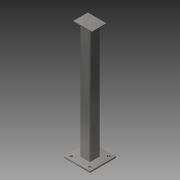
# Autodesk Inventor part: Ст1 - Metal rack
Saved by Autodesk Inventor 2020.1 (Build 241239000, 239)
## iProperties
Created: 2017-07-27
Part Number: Ст1 - Metal rack
Material: Сталь, углеродистая
Document SubType Name: Modeling
Designer: Головченко
Density: 7.87 g/cm^3
Appearance: Сталь — полированная
Mass&: 0
Author: Головченко
Autodesk Inventor part; units mm, degrees
(part 1 of 4)
ref_plane "YZ Plane" through (0, 0, 0) normal (1, 0, 0) x (0, 1, 0)
ref_plane "XZ Plane" through (0, 0, 0) normal (0, 1, 0) x (-1, 0, 0)
ref_plane "XY Plane" through (0, 0, 0) normal (0, 0, 1) x (1, 0, 0)
sketch "Кутник 20х3" plane through (0, 0, 0) normal (0, 0, 1) x (1, 0, 0)
  line L0 (0, 0) -> (0, 20)
  line L1 (0, 20) -> (1.8, 20)
  arc A0 (3, 18.8) -> (1.8, 20) centre (1.8, 18.8) ccw
  line L2 (3, 18.8) -> (3, 6.5)
  arc A1 (3, 6.5) -> (6.5, 3) centre (6.5, 6.5) ccw
  line L3 (6.5, 3) -> (18.8, 3)
  arc A2 (20, 1.8) -> (18.8, 3) centre (18.8, 1.8) ccw
  line L4 (20, 1.8) -> (20, 0)
  line L5 (20, 0) -> (0, 0)
  point P0 (8.2133, 8.2133)
  dimension "d0" = 20
  dimension "d1" = 3
  dimension "d2" = 3.5
  dimension "d3" = 1.2
  measures "d0" distance between parallel lines of L5 L1
  measures "d1" distance between parallel lines of L5 L3
  measures "d2" radius of A1
  measures "d3" radius of A2
sketch "Кутник 20х4" plane through (0, 0, 0) normal (0, 0, 1) x (1, 0, 0)
  line L0 (4.9813, 3.7617) -> (4.9813, 23.7617)
  line L1 (4.9813, 23.7617) -> (7.7813, 23.7617)
  arc A0 (8.9813, 22.5617) -> (7.7813, 23.7617) centre (7.7813, 22.5617) ccw
  line L2 (8.9813, 22.5617) -> (8.9813, 11.2617)
  arc A1 (8.9813, 11.2617) -> (12.4813, 7.7617) centre (12.4813, 11.2617) ccw
  line L3 (12.4813, 7.7617) -> (23.7813, 7.7617)
  arc A2 (24.9813, 6.5617) -> (23.7813, 7.7617) centre (23.7813, 6.5617) ccw
  line L4 (24.9813, 6.5617) -> (24.9813, 3.7617)
  line L5 (24.9813, 3.7617) -> (4.9813, 3.7617)
  point P0 (8.2133, 8.2133)
  dimension "d4" = 20
  dimension "d5" = 4
  dimension "d6" = 3.5
  dimension "d7" = 1.2
  measures "d4" distance between parallel lines of L5 L1
  measures "d5" distance between parallel lines of L5 L3
  measures "d6" radius of A1
  measures "d7" radius of A2
sketch "Кутник 25х3" plane through (0, 0, 0) normal (0, 0, 1) x (1, 0, 0)
  line L0 (0, 0) -> (0, 25)
  line L1 (0, 25) -> (1.8, 25)
  arc A0 (3, 23.8) -> (1.8, 25) centre (1.8, 23.8) ccw
  line L2 (3, 23.8) -> (3, 6.5)
  arc A1 (3, 6.5) -> (6.5, 3) centre (6.5, 6.5) ccw
  line L3 (6.5, 3) -> (23.8, 3)
  arc A2 (25, 1.8) -> (23.8, 3) centre (23.8, 1.8) ccw
  line L4 (25, 1.8) -> (25, 0)
  line L5 (25, 0) -> (0, 0)
  point P0 (8.2133, 8.2133)
  dimension "d8" = 25
  dimension "d9" = 3
  dimension "d10" = 3.5
  dimension "d11" = 1.2
  measures "d8" distance between parallel lines of L5 L1
  measures "d9" distance between parallel lines of L5 L3
  measures "d10" radius of A1
  measures "d11" radius of A2
sketch "Кутник 25х4" plane through (0, 0, 0) normal (0, 0, 1) x (1, 0, 0)
  line L0 (2.773, 6.781) -> (2.773, 31.781)
  line L1 (2.773, 31.781) -> (5.573, 31.781)
  arc A0 (6.773, 30.581) -> (5.573, 31.781) centre (5.573, 30.581) ccw
  line L2 (6.773, 30.581) -> (6.773, 14.281)
  arc A1 (6.773, 14.281) -> (10.273, 10.781) centre (10.273, 14.281) ccw
  line L3 (10.273, 10.781) -> (26.573, 10.781)
  arc A2 (27.773, 9.581) -> (26.573, 10.781) centre (26.573, 9.581) ccw
  line L4 (27.773, 9.581) -> (27.773, 6.781)
  line L5 (27.773, 6.781) -> (2.773, 6.781)
  point P0 (8.2133, 8.2133)
  dimension "d12" = 25
  dimension "d13" = 4
  dimension "d14" = 3.5
  dimension "d15" = 1.2
  measures "d12" distance between parallel lines of L5 L1
  measures "d13" distance between parallel lines of L5 L3
  measures "d14" radius of A1
  measures "d15" radius of A2
sketch "Кутник 28х3" plane through (0, 0, 0) normal (0, 0, 1) x (1, 0, 0)
  line L0 (4.3504, 3.0393) -> (4.3504, 31.0393)
  line L1 (4.3504, 31.0393) -> (6.0504, 31.0393)
  arc A0 (7.3504, 29.7393) -> (6.0504, 31.0393) centre (6.0504, 29.7393) ccw
  line L2 (7.3504, 29.7393) -> (7.3504, 10.0393)
  arc A1 (7.3504, 10.0393) -> (11.3504, 6.0393) centre (11.3504, 10.0393) ccw
  line L3 (11.3504, 6.0393) -> (31.0504, 6.0393)
  arc A2 (32.3504, 4.7393) -> (31.0504, 6.0393) centre (31.0504, 4.7393) ccw
  line L4 (32.3504, 4.7393) -> (32.3504, 3.0393)
  line L5 (32.3504, 3.0393) -> (4.3504, 3.0393)
  point P0 (8.2133, 8.2133)
  dimension "d16" = 28
  dimension "d17" = 3
  dimension "d18" = 4
  dimension "d19" = 1.3
  measures "d16" distance between parallel lines of L5 L1
  measures "d17" distance between parallel lines of L5 L3
  measures "d18" radius of A1
  measures "d19" radius of A2
sketch "Кутник 32х3" plane through (0, 0, 0) normal (0, 0, 1) x (1, 0, 0)
  line L0 (2.7965, 1.5965) -> (2.7965, 33.5965)
  line L1 (2.7965, 33.5965) -> (4.2965, 33.5965)
  arc A0 (5.7965, 32.0965) -> (4.2965, 33.5965) centre (4.2965, 32.0965) ccw
  line L2 (5.7965, 32.0965) -> (5.7965, 9.0965)
  arc A1 (5.7965, 9.0965) -> (10.2965, 4.5965) centre (10.2965, 9.0965) ccw
  line L3 (10.2965, 4.5965) -> (33.2965, 4.5965)
  arc A2 (34.7965, 3.0965) -> (33.2965, 4.5965) centre (33.2965, 3.0965) ccw
  line L4 (34.7965, 3.0965) -> (34.7965, 1.5965)
  line L5 (34.7965, 1.5965) -> (2.7965, 1.5965)
  point P0 (8.2133, 8.2133)
  dimension "d20" = 32
  dimension "d21" = 3
  dimension "d22" = 4.5
  dimension "d23" = 1.5
  measures "d20" distance between parallel lines of L5 L1
  measures "d21" distance between parallel lines of L5 L3
  measures "d22" radius of A1
  measures "d23" radius of A2
sketch "Кутник 32х4" plane through (0, 0, 0) normal (0, 0, 1) x (1, 0, 0)
  line L0 (2.2581, 1.0965) -> (2.2581, 33.0965)
  line L1 (2.2581, 33.0965) -> (4.7581, 33.0965)
  arc A0 (6.2581, 31.5965) -> (4.7581, 33.0965) centre (4.7581, 31.5965) ccw
  line L2 (6.2581, 31.5965) -> (6.2581, 9.5965)
  arc A1 (6.2581, 9.5965) -> (10.7581, 5.0965) centre (10.7581, 9.5965) ccw
  line L3 (10.7581, 5.0965) -> (32.7581, 5.0965)
  arc A2 (34.2581, 3.5965) -> (32.7581, 5.0965) centre (32.7581, 3.5965) ccw
  line L4 (34.2581, 3.5965) -> (34.2581, 1.0965)
  line L5 (34.2581, 1.0965) -> (2.2581, 1.0965)
  point P0 (8.2133, 8.2133)
  dimension "d24" = 32
  dimension "d25" = 4
  dimension "d26" = 4.5
  dimension "d27" = 1.5
  measures "d24" distance between parallel lines of L5 L1
  measures "d25" distance between parallel lines of L5 L3
  measures "d26" radius of A1
  measures "d27" radius of A2
sketch "Кутник 36х3" plane through (0, 0, 0) normal (0, 0, 1) x (1, 0, 0)
  line L0 (1.2581, 0.1679) -> (1.2581, 36.1679)
  line L1 (1.2581, 36.1679) -> (2.7581, 36.1679)
  arc A0 (4.2581, 34.6679) -> (2.7581, 36.1679) centre (2.7581, 34.6679) ccw
  line L2 (4.2581, 34.6679) -> (4.2581, 7.6679)
  arc A1 (4.2581, 7.6679) -> (8.7581, 3.1679) centre (8.7581, 7.6679) ccw
  line L3 (8.7581, 3.1679) -> (35.7581, 3.1679)
  arc A2 (37.2581, 1.6679) -> (35.7581, 3.1679) centre (35.7581, 1.6679) ccw
  line L4 (37.2581, 1.6679) -> (37.2581, 0.1679)
  line L5 (37.2581, 0.1679) -> (1.2581, 0.1679)
  point P0 (8.2133, 8.2133)
  dimension "d28" = 36
  dimension "d29" = 3
  dimension "d30" = 4.5
  dimension "d31" = 1.5
  measures "d28" distance between parallel lines of L5 L1
  measures "d29" distance between parallel lines of L5 L3
  measures "d30" radius of A1
  measures "d31" radius of A2
sketch "Кутник 36х4" plane through (0, 0, 0) normal (0, 0, 1) x (1, 0, 0)
  line L0 (0.7196, -0.3321) -> (0.7196, 35.6679)
  line L1 (0.7196, 35.6679) -> (3.2196, 35.6679)
  arc A0 (4.7196, 34.1679) -> (3.2196, 35.6679) centre (3.2196, 34.1679) ccw
  line L2 (4.7196, 34.1679) -> (4.7196, 8.1679)
  arc A1 (4.7196, 8.1679) -> (9.2196, 3.6679) centre (9.2196, 8.1679) ccw
  line L3 (9.2196, 3.6679) -> (35.2196, 3.6679)
  arc A2 (36.7196, 2.1679) -> (35.2196, 3.6679) centre (35.2196, 2.1679) ccw
  line L4 (36.7196, 2.1679) -> (36.7196, -0.3321)
  line L5 (36.7196, -0.3321) -> (0.7196, -0.3321)
  point P0 (8.2133, 8.2133)
  dimension "d32" = 36
  dimension "d33" = 4
  dimension "d34" = 4.5
  dimension "d35" = 1.5
  measures "d32" distance between parallel lines of L5 L1
  measures "d33" distance between parallel lines of L5 L3
  measures "d34" radius of A1
  measures "d35" radius of A2
sketch "Кутник 40х3" plane through (0, 0, 0) normal (0, 0, 1) x (1, 0, 0)
  line L0 (-0.2958, -1.275) -> (-0.2958, 38.725)
  line L1 (-0.2958, 38.725) -> (1.0042, 38.725)
  arc A0 (2.7042, 37.025) -> (1.0042, 38.725) centre (1.0042, 37.025) ccw
  line L2 (2.7042, 37.025) -> (2.7042, 6.725)
  arc A1 (2.7042, 6.725) -> (7.7042, 1.725) centre (7.7042, 6.725) ccw
  line L3 (7.7042, 1.725) -> (38.0042, 1.725)
  arc A2 (39.7042, 0.025) -> (38.0042, 1.725) centre (38.0042, 0.025) ccw
  line L4 (39.7042, 0.025) -> (39.7042, -1.275)
  line L5 (39.7042, -1.275) -> (-0.2958, -1.275)
  point P0 (8.2133, 8.2133)
  dimension "d36" = 40
  dimension "d37" = 3
  dimension "d38" = 5
  dimension "d39" = 1.7
  measures "d36" distance between parallel lines of L5 L1
  measures "d37" distance between parallel lines of L5 L3
  measures "d38" radius of A1
  measures "d39" radius of A2
sketch "Кутник 40х4" plane through (0, 0, 0) normal (0, 0, 1) x (1, 0, 0)
  line L0 (-0.8342, -1.775) -> (-0.8342, 38.225)
  line L1 (-0.8342, 38.225) -> (1.4658, 38.225)
  arc A0 (3.1658, 36.525) -> (1.4658, 38.225) centre (1.4658, 36.525) ccw
  line L2 (3.1658, 36.525) -> (3.1658, 7.225)
  arc A1 (3.1658, 7.225) -> (8.1658, 2.225) centre (8.1658, 7.225) ccw
  line L3 (8.1658, 2.225) -> (37.4658, 2.225)
  arc A2 (39.1658, 0.525) -> (37.4658, 2.225) centre (37.4658, 0.525) ccw
  line L4 (39.1658, 0.525) -> (39.1658, -1.775)
  line L5 (39.1658, -1.775) -> (-0.8342, -1.775)
  point P0 (8.2133, 8.2133)
  dimension "d40" = 40
  dimension "d41" = 4
  dimension "d42" = 5
  dimension "d43" = 1.7
  measures "d40" distance between parallel lines of L5 L1
  measures "d41" distance between parallel lines of L5 L3
  measures "d42" radius of A1
  measures "d43" radius of A2
sketch "Кутник 40х5" plane through (0, 0, 0) normal (0, 0, 1) x (1, 0, 0)
  line L0 (-1.3727, -2.275) -> (-1.3727, 37.725)
  line L1 (-1.3727, 37.725) -> (1.9273, 37.725)
  arc A0 (3.6273, 36.025) -> (1.9273, 37.725) centre (1.9273, 36.025) ccw
  line L2 (3.6273, 36.025) -> (3.6273, 7.725)
  arc A1 (3.6273, 7.725) -> (8.6273, 2.725) centre (8.6273, 7.725) ccw
  line L3 (8.6273, 2.725) -> (36.9273, 2.725)
  arc A2 (38.6273, 1.025) -> (36.9273, 2.725) centre (36.9273, 1.025) ccw
  line L4 (38.6273, 1.025) -> (38.6273, -2.275)
  line L5 (38.6273, -2.275) -> (-1.3727, -2.275)
  point P0 (8.2133, 8.2133)
  dimension "d44" = 40
  dimension "d45" = 5
  dimension "d46" = 5
  dimension "d47" = 1.7
  measures "d44" distance between parallel lines of L5 L1
  measures "d45" distance between parallel lines of L5 L3
  measures "d46" radius of A1
  measures "d47" radius of A2
sketch "Кутник 45х3" plane through (0, 0, 0) normal (0, 0, 1) x (1, 0, 0)
  line L0 (-2.2188, -3.0607) -> (-2.2188, 41.9393)
  line L1 (-2.2188, 41.9393) -> (-0.9188, 41.9393)
  arc A0 (0.7812, 40.2393) -> (-0.9188, 41.9393) centre (-0.9188, 40.2393) ccw
  line L2 (0.7812, 40.2393) -> (0.7812, 4.9393)
  arc A1 (0.7812, 4.9393) -> (5.7812, -0.0607) centre (5.7812, 4.9393) ccw
  line L3 (5.7812, -0.0607) -> (41.0812, -0.0607)
  arc A2 (42.7812, -1.7607) -> (41.0812, -0.0607) centre (41.0812, -1.7607) ccw
  line L4 (42.7812, -1.7607) -> (42.7812, -3.0607)
  line L5 (42.7812, -3.0607) -> (-2.2188, -3.0607)
  point P0 (8.2133, 8.2133)
  dimension "d48" = 45
  dimension "d49" = 3
  dimension "d50" = 5
  dimension "d51" = 1.7
  measures "d48" distance between parallel lines of L5 L1
  measures "d49" distance between parallel lines of L5 L3
  measures "d50" radius of A1
  measures "d51" radius of A2
sketch "Кутник 45х4" plane through (0, 0, 0) normal (0, 0, 1) x (1, 0, 0)
  line L0 (-2.7573, -3.5607) -> (-2.7573, 41.4393)
  line L1 (-2.7573, 41.4393) -> (-0.4573, 41.4393)
  arc A0 (1.2427, 39.7393) -> (-0.4573, 41.4393) centre (-0.4573, 39.7393) ccw
  line L2 (1.2427, 39.7393) -> (1.2427, 5.4393)
  arc A1 (1.2427, 5.4393) -> (6.2427, 0.4393) centre (6.2427, 5.4393) ccw
  line L3 (6.2427, 0.4393) -> (40.5427, 0.4393)
  arc A2 (42.2427, -1.2607) -> (40.5427, 0.4393) centre (40.5427, -1.2607) ccw
  line L4 (42.2427, -1.2607) -> (42.2427, -3.5607)
  line L5 (42.2427, -3.5607) -> (-2.7573, -3.5607)
  point P0 (8.2133, 8.2133)
  dimension "d52" = 45
  dimension "d53" = 4
  dimension "d54" = 5
  dimension "d55" = 1.7
  measures "d52" distance between parallel lines of L5 L1
  measures "d53" distance between parallel lines of L5 L3
  measures "d54" radius of A1
  measures "d55" radius of A2
sketch "Кутник 45х5" plane through (0, 0, 0) normal (0, 0, 1) x (1, 0, 0)
  line L0 (-3.2958, -4.0607) -> (-3.2958, 40.9393)
  line L1 (-3.2958, 40.9393) -> (0.0042, 40.9393)
  arc A0 (1.7042, 39.2393) -> (0.0042, 40.9393) centre (0.0042, 39.2393) ccw
  line L2 (1.7042, 39.2393) -> (1.7042, 5.9393)
  arc A1 (1.7042, 5.9393) -> (6.7042, 0.9393) centre (6.7042, 5.9393) ccw
  line L3 (6.7042, 0.9393) -> (40.0042, 0.9393)
  arc A2 (41.7042, -0.7607) -> (40.0042, 0.9393) centre (40.0042, -0.7607) ccw
  line L4 (41.7042, -0.7607) -> (41.7042, -4.0607)
  line L5 (41.7042, -4.0607) -> (-3.2958, -4.0607)
  point P0 (8.2133, 8.2133)
  dimension "d56" = 45
  dimension "d57" = 5
  dimension "d58" = 5
  dimension "d59" = 1.7
  measures "d56" distance between parallel lines of L5 L1
  measures "d57" distance between parallel lines of L5 L3
  measures "d58" radius of A1
  measures "d59" radius of A2
sketch "Кутник 50х3" plane through (0, 0, 0) normal (0, 0, 1) x (1, 0, 0)
  line L0 (-4.1881, -4.8892) -> (-4.1881, 45.1108)
  line L1 (-4.1881, 45.1108) -> (-2.9881, 45.1108)
  arc A0 (-1.1881, 43.3108) -> (-2.9881, 45.1108) centre (-2.9881, 43.3108) ccw
  line L2 (-1.1881, 43.3108) -> (-1.1881, 3.6108)
  arc A1 (-1.1881, 3.6108) -> (4.3119, -1.8892) centre (4.3119, 3.6108) ccw
  line L3 (4.3119, -1.8892) -> (44.0119, -1.8892)
  arc A2 (45.8119, -3.6892) -> (44.0119, -1.8892) centre (44.0119, -3.6892) ccw
  line L4 (45.8119, -3.6892) -> (45.8119, -4.8892)
  line L5 (45.8119, -4.8892) -> (-4.1881, -4.8892)
  point P0 (8.2133, 8.2133)
  dimension "d60" = 50
  dimension "d61" = 3
  dimension "d62" = 5.5
  dimension "d63" = 1.8
  measures "d60" distance between parallel lines of L5 L1
  measures "d61" distance between parallel lines of L5 L3
  measures "d62" radius of A1
  measures "d63" radius of A2
sketch "Кутник 50х4" plane through (0, 0, 0) normal (0, 0, 1) x (1, 0, 0)
  line L0 (-4.7265, -5.3892) -> (-4.7265, 44.6108)
  line L1 (-4.7265, 44.6108) -> (-2.5265, 44.6108)
  arc A0 (-0.7265, 42.8108) -> (-2.5265, 44.6108) centre (-2.5265, 42.8108) ccw
  line L2 (-0.7265, 42.8108) -> (-0.7265, 4.1108)
  arc A1 (-0.7265, 4.1108) -> (4.7735, -1.3892) centre (4.7735, 4.1108) ccw
  line L3 (4.7735, -1.3892) -> (43.4735, -1.3892)
  arc A2 (45.2735, -3.1892) -> (43.4735, -1.3892) centre (43.4735, -3.1892) ccw
  line L4 (45.2735, -3.1892) -> (45.2735, -5.3892)
  line L5 (45.2735, -5.3892) -> (-4.7265, -5.3892)
  point P0 (8.2133, 8.2133)
  dimension "d64" = 50
  dimension "d65" = 4
  dimension "d66" = 5.5
  dimension "d67" = 1.8
  measures "d64" distance between parallel lines of L5 L1
  measures "d65" distance between parallel lines of L5 L3
  measures "d66" radius of A1
  measures "d67" radius of A2
sketch "Кутник 50х5" plane through (0, 0, 0) normal (0, 0, 1) x (1, 0, 0)
  line L0 (-5.265, -5.8892) -> (-5.265, 44.1108)
  line L1 (-5.265, 44.1108) -> (-2.065, 44.1108)
  arc A0 (-0.265, 42.3108) -> (-2.065, 44.1108) centre (-2.065, 42.3108) ccw
  line L2 (-0.265, 42.3108) -> (-0.265, 4.6108)
  arc A1 (-0.265, 4.6108) -> (5.235, -0.8892) centre (5.235, 4.6108) ccw
  line L3 (5.235, -0.8892) -> (42.935, -0.8892)
  arc A2 (44.735, -2.6892) -> (42.935, -0.8892) centre (42.935, -2.6892) ccw
  line L4 (44.735, -2.6892) -> (44.735, -5.8892)
  line L5 (44.735, -5.8892) -> (-5.265, -5.8892)
  point P0 (8.2133, 8.2133)
  dimension "d68" = 50
  dimension "d69" = 5
  dimension "d70" = 5.5
  dimension "d71" = 1.8
  measures "d68" distance between parallel lines of L5 L1
  measures "d69" distance between parallel lines of L5 L3
  measures "d70" radius of A1
  measures "d71" radius of A2
sketch "Кутник 56х4" plane through (0, 0, 0) normal (0, 0, 1) x (1, 0, 0)
  line L0 (-7.0496, -7.5464) -> (-7.0496, 48.4536)
  line L1 (-7.0496, 48.4536) -> (-5.0496, 48.4536)
  arc A0 (-3.0496, 46.4536) -> (-5.0496, 48.4536) centre (-5.0496, 46.4536) ccw
  line L2 (-3.0496, 46.4536) -> (-3.0496, 2.4536)
  arc A1 (-3.0496, 2.4536) -> (2.9504, -3.5464) centre (2.9504, 2.4536) ccw
  line L3 (2.9504, -3.5464) -> (46.9504, -3.5464)
  arc A2 (48.9504, -5.5464) -> (46.9504, -3.5464) centre (46.9504, -5.5464) ccw
  line L4 (48.9504, -5.5464) -> (48.9504, -7.5464)
  line L5 (48.9504, -7.5464) -> (-7.0496, -7.5464)
  point P0 (8.2133, 8.2133)
  dimension "d72" = 56
  dimension "d73" = 4
  dimension "d74" = 6
  dimension "d75" = 2
  measures "d72" distance between parallel lines of L5 L1
  measures "d73" distance between parallel lines of L5 L3
  measures "d74" radius of A1
  measures "d75" radius of A2
sketch "Кутник 56х5" plane through (0, 0, 0) normal (0, 0, 1) x (1, 0, 0)
  line L0 (-7.5881, -8.0464) -> (-7.5881, 47.9536)
  line L1 (-7.5881, 47.9536) -> (-4.5881, 47.9536)
  arc A0 (-2.5881, 45.9536) -> (-4.5881, 47.9536) centre (-4.5881, 45.9536) ccw
  line L2 (-2.5881, 45.9536) -> (-2.5881, 2.9536)
  arc A1 (-2.5881, 2.9536) -> (3.4119, -3.0464) centre (3.4119, 2.9536) ccw
  line L3 (3.4119, -3.0464) -> (46.4119, -3.0464)
  arc A2 (48.4119, -5.0464) -> (46.4119, -3.0464) centre (46.4119, -5.0464) ccw
  line L4 (48.4119, -5.0464) -> (48.4119, -8.0464)
  line L5 (48.4119, -8.0464) -> (-7.5881, -8.0464)
  point P0 (8.2133, 8.2133)
  dimension "d76" = 56
  dimension "d77" = 5
  dimension "d78" = 6
  dimension "d79" = 2
  measures "d76" distance between parallel lines of L5 L1
  measures "d77" distance between parallel lines of L5 L3
  measures "d78" radius of A1
  measures "d79" radius of A2
sketch "Кутник 63х4" plane through (0, 0, 0) normal (0, 0, 1) x (1, 0, 0)
  line L0 (-9.8035, -10.1035) -> (-9.8035, 52.8965)
  line L1 (-9.8035, 52.8965) -> (-8.1035, 52.8965)
  arc A0 (-5.8035, 50.5965) -> (-8.1035, 52.8965) centre (-8.1035, 50.5965) ccw
  line L2 (-5.8035, 50.5965) -> (-5.8035, 0.8965)
  arc A1 (-5.8035, 0.8965) -> (1.1965, -6.1035) centre (1.1965, 0.8965) ccw
  line L3 (1.1965, -6.1035) -> (50.8965, -6.1035)
  arc A2 (53.1965, -8.4035) -> (50.8965, -6.1035) centre (50.8965, -8.4035) ccw
  line L4 (53.1965, -8.4035) -> (53.1965, -10.1035)
  line L5 (53.1965, -10.1035) -> (-9.8035, -10.1035)
  point P0 (8.2133, 8.2133)
  dimension "d80" = 63
  dimension "d81" = 4
  dimension "d82" = 7
  dimension "d83" = 2.3
  measures "d80" distance between parallel lines of L5 L1
  measures "d81" distance between parallel lines of L5 L3
  measures "d82" radius of A1
  measures "d83" radius of A2
sketch "Кутник 63х5" plane through (0, 0, 0) normal (0, 0, 1) x (1, 0, 0)
  line L0 (-10.3419, -10.6035) -> (-10.3419, 52.3965)
  line L1 (-10.3419, 52.3965) -> (-7.6419, 52.3965)
  arc A0 (-5.3419, 50.0965) -> (-7.6419, 52.3965) centre (-7.6419, 50.0965) ccw
  line L2 (-5.3419, 50.0965) -> (-5.3419, 1.3965)
  arc A1 (-5.3419, 1.3965) -> (1.6581, -5.6035) centre (1.6581, 1.3965) ccw
  line L3 (1.6581, -5.6035) -> (50.3581, -5.6035)
  arc A2 (52.6581, -7.9035) -> (50.3581, -5.6035) centre (50.3581, -7.9035) ccw
  line L4 (52.6581, -7.9035) -> (52.6581, -10.6035)
  line L5 (52.6581, -10.6035) -> (-10.3419, -10.6035)
  point P0 (8.2133, 8.2133)
  dimension "d84" = 63
  dimension "d85" = 5
  dimension "d86" = 7
  dimension "d87" = 2.3
  measures "d84" distance between parallel lines of L5 L1
  measures "d85" distance between parallel lines of L5 L3
  measures "d86" radius of A1
  measures "d87" radius of A2
sketch "Кутник 63х6" plane through (0, 0, 0) normal (0, 0, 1) x (1, 0, 0)
  line L0 (-10.8804, -11.1035) -> (-10.8804, 51.8965)
  line L1 (-10.8804, 51.8965) -> (-7.1804, 51.8965)
  arc A0 (-4.8804, 49.5965) -> (-7.1804, 51.8965) centre (-7.1804, 49.5965) ccw
  line L2 (-4.8804, 49.5965) -> (-4.8804, 1.8965)
  arc A1 (-4.8804, 1.8965) -> (2.1196, -5.1035) centre (2.1196, 1.8965) ccw
  line L3 (2.1196, -5.1035) -> (49.8196, -5.1035)
  arc A2 (52.1196, -7.4035) -> (49.8196, -5.1035) centre (49.8196, -7.4035) ccw
  line L4 (52.1196, -7.4035) -> (52.1196, -11.1035)
  line L5 (52.1196, -11.1035) -> (-10.8804, -11.1035)
  point P0 (8.2133, 8.2133)
  dimension "d88" = 63
  dimension "d89" = 6
  dimension "d90" = 7
  dimension "d91" = 2.3
  measures "d88" distance between parallel lines of L5 L1
  measures "d89" distance between parallel lines of L5 L3
  measures "d90" radius of A1
  measures "d91" radius of A2
sketch "Кутник 70х4.5" plane through (0, 0, 0) normal (0, 0, 1) x (1, 0, 0)
  line L0 (-12.7958, -12.8821) -> (-12.7958, 57.1179)
  line L1 (-12.7958, 57.1179) -> (-10.9958, 57.1179)
  arc A0 (-8.2958, 54.4179) -> (-10.9958, 57.1179) centre (-10.9958, 54.4179) ccw
  line L2 (-8.2958, 54.4179) -> (-8.2958, -0.3821)
  arc A1 (-8.2958, -0.3821) -> (-0.2958, -8.3821) centre (-0.2958, -0.3821) ccw
  line L3 (-0.2958, -8.3821) -> (54.5042, -8.3821)
  arc A2 (57.2042, -11.0821) -> (54.5042, -8.3821) centre (54.5042, -11.0821) ccw
  line L4 (57.2042, -11.0821) -> (57.2042, -12.8821)
  line L5 (57.2042, -12.8821) -> (-12.7958, -12.8821)
  point P0 (8.2133, 8.2133)
  dimension "d92" = 70
  dimension "d93" = 4.5
  dimension "d94" = 8
  dimension "d95" = 2.7
  measures "d92" distance between parallel lines of L5 L1
  measures "d93" distance between parallel lines of L5 L3
  measures "d94" radius of A1
  measures "d95" radius of A2
sketch "Кутник 70х5" plane through (0, 0, 0) normal (0, 0, 1) x (1, 0, 0)
  line L0 (-13.065, -13.1321) -> (-13.065, 56.8679)
  line L1 (-13.065, 56.8679) -> (-10.765, 56.8679)
  arc A0 (-8.065, 54.1679) -> (-10.765, 56.8679) centre (-10.765, 54.1679) ccw
  line L2 (-8.065, 54.1679) -> (-8.065, -0.1321)
  arc A1 (-8.065, -0.1321) -> (-0.065, -8.1321) centre (-0.065, -0.1321) ccw
  line L3 (-0.065, -8.1321) -> (54.235, -8.1321)
  arc A2 (56.935, -10.8321) -> (54.235, -8.1321) centre (54.235, -10.8321) ccw
  line L4 (56.935, -10.8321) -> (56.935, -13.1321)
  line L5 (56.935, -13.1321) -> (-13.065, -13.1321)
  point P0 (8.2133, 8.2133)
  dimension "d96" = 70
  dimension "d97" = 5
  dimension "d98" = 8
  dimension "d99" = 2.7
  measures "d96" distance between parallel lines of L5 L1
  measures "d97" distance between parallel lines of L5 L3
  measures "d98" radius of A1
  measures "d99" radius of A2
sketch "Кутник 70х6" plane through (0, 0, 0) normal (0, 0, 1) x (1, 0, 0)
  line L0 (-13.6035, -13.6321) -> (-13.6035, 56.3679)
  line L1 (-13.6035, 56.3679) -> (-10.3035, 56.3679)
  arc A0 (-7.6035, 53.6679) -> (-10.3035, 56.3679) centre (-10.3035, 53.6679) ccw
  line L2 (-7.6035, 53.6679) -> (-7.6035, 0.3679)
  arc A1 (-7.6035, 0.3679) -> (0.3965, -7.6321) centre (0.3965, 0.3679) ccw
  line L3 (0.3965, -7.6321) -> (53.6965, -7.6321)
  arc A2 (56.3965, -10.3321) -> (53.6965, -7.6321) centre (53.6965, -10.3321) ccw
  line L4 (56.3965, -10.3321) -> (56.3965, -13.6321)
  line L5 (56.3965, -13.6321) -> (-13.6035, -13.6321)
  point P0 (8.2133, 8.2133)
  dimension "d100" = 70
  dimension "d101" = 6
  dimension "d102" = 8
  dimension "d103" = 2.7
  measures "d100" distance between parallel lines of L5 L1
  measures "d101" distance between parallel lines of L5 L3
  measures "d102" radius of A1
  measures "d103" radius of A2
sketch "Кутник 70х7" plane through (0, 0, 0) normal (0, 0, 1) x (1, 0, 0)
  line L0 (-14.1419, -14.1321) -> (-14.1419, 55.8679)
  line L1 (-14.1419, 55.8679) -> (-9.8419, 55.8679)
  arc A0 (-7.1419, 53.1679) -> (-9.8419, 55.8679) centre (-9.8419, 53.1679) ccw
  line L2 (-7.1419, 53.1679) -> (-7.1419, 0.8679)
  arc A1 (-7.1419, 0.8679) -> (0.8581, -7.1321) centre (0.8581, 0.8679) ccw
  line L3 (0.8581, -7.1321) -> (53.1581, -7.1321)
  arc A2 (55.8581, -9.8321) -> (53.1581, -7.1321) centre (53.1581, -9.8321) ccw
  line L4 (55.8581, -9.8321) -> (55.8581, -14.1321)
  line L5 (55.8581, -14.1321) -> (-14.1419, -14.1321)
  point P0 (8.2133, 8.2133)
  dimension "d104" = 70
  dimension "d105" = 7
  dimension "d106" = 8
  dimension "d107" = 2.7
  measures "d104" distance between parallel lines of L5 L1
  measures "d105" distance between parallel lines of L5 L3
  measures "d106" radius of A1
  measures "d107" radius of A2
sketch "Кутник 70х8" plane through (0, 0, 0) normal (0, 0, 1) x (1, 0, 0)
  line L0 (-14.6804, -14.6321) -> (-14.6804, 55.3679)
  line L1 (-14.6804, 55.3679) -> (-9.3804, 55.3679)
  arc A0 (-6.6804, 52.6679) -> (-9.3804, 55.3679) centre (-9.3804, 52.6679) ccw
  line L2 (-6.6804, 52.6679) -> (-6.6804, 1.3679)
  arc A1 (-6.6804, 1.3679) -> (1.3196, -6.6321) centre (1.3196, 1.3679) ccw
  line L3 (1.3196, -6.6321) -> (52.6196, -6.6321)
  arc A2 (55.3196, -9.3321) -> (52.6196, -6.6321) centre (52.6196, -9.3321) ccw
  line L4 (55.3196, -9.3321) -> (55.3196, -14.6321)
  line L5 (55.3196, -14.6321) -> (-14.6804, -14.6321)
  point P0 (8.2133, 8.2133)
  dimension "d108" = 70
  dimension "d109" = 8
  dimension "d110" = 8
  dimension "d111" = 2.7
  measures "d108" distance between parallel lines of L5 L1
  measures "d109" distance between parallel lines of L5 L3
  measures "d110" radius of A1
  measures "d111" radius of A2
sketch "Кутник 75х5" plane through (0, 0, 0) normal (0, 0, 1) x (1, 0, 0)
  line L0 (-15.0496, -14.975) -> (-15.0496, 60.025)
  line L1 (-15.0496, 60.025) -> (-13.0496, 60.025)
  arc A0 (-10.0496, 57.025) -> (-13.0496, 60.025) centre (-13.0496, 57.025) ccw
  line L2 (-10.0496, 57.025) -> (-10.0496, -0.975)
  arc A1 (-10.0496, -0.975) -> (-1.0496, -9.975) centre (-1.0496, -0.975) ccw
  line L3 (-1.0496, -9.975) -> (56.9504, -9.975)
  arc A2 (59.9504, -12.975) -> (56.9504, -9.975) centre (56.9504, -12.975) ccw
  line L4 (59.9504, -12.975) -> (59.9504, -14.975)
  line L5 (59.9504, -14.975) -> (-15.0496, -14.975)
  point P0 (8.2133, 8.2133)
  dimension "d112" = 75
  dimension "d113" = 5
  dimension "d114" = 9
  dimension "d115" = 3
  measures "d112" distance between parallel lines of L5 L1
  measures "d113" distance between parallel lines of L5 L3
  measures "d114" radius of A1
  measures "d115" radius of A2
sketch "Кутник 75х6" plane through (0, 0, 0) normal (0, 0, 1) x (1, 0, 0)
  line L0 (-15.5881, -15.475) -> (-15.5881, 59.525)
  line L1 (-15.5881, 59.525) -> (-12.5881, 59.525)
  arc A0 (-9.5881, 56.525) -> (-12.5881, 59.525) centre (-12.5881, 56.525) ccw
  line L2 (-9.5881, 56.525) -> (-9.5881, -0.475)
  arc A1 (-9.5881, -0.475) -> (-0.5881, -9.475) centre (-0.5881, -0.475) ccw
  line L3 (-0.5881, -9.475) -> (56.4119, -9.475)
  arc A2 (59.4119, -12.475) -> (56.4119, -9.475) centre (56.4119, -12.475) ccw
  line L4 (59.4119, -12.475) -> (59.4119, -15.475)
  line L5 (59.4119, -15.475) -> (-15.5881, -15.475)
  point P0 (8.2133, 8.2133)
  dimension "d116" = 75
  dimension "d117" = 6
  dimension "d118" = 9
  dimension "d119" = 3
  measures "d116" distance between parallel lines of L5 L1
  measures "d117" distance between parallel lines of L5 L3
  measures "d118" radius of A1
  measures "d119" radius of A2
sketch "Кутник 75х7" plane through (0, 0, 0) normal (0, 0, 1) x (1, 0, 0)
  line L0 (-16.1265, -15.975) -> (-16.1265, 59.025)
  line L1 (-16.1265, 59.025) -> (-12.1265, 59.025)
  arc A0 (-9.1265, 56.025) -> (-12.1265, 59.025) centre (-12.1265, 56.025) ccw
  line L2 (-9.1265, 56.025) -> (-9.1265, 0.025)
  arc A1 (-9.1265, 0.025) -> (-0.1265, -8.975) centre (-0.1265, 0.025) ccw
  line L3 (-0.1265, -8.975) -> (55.8735, -8.975)
  arc A2 (58.8735, -11.975) -> (55.8735, -8.975) centre (55.8735, -11.975) ccw
  line L4 (58.8735, -11.975) -> (58.8735, -15.975)
  line L5 (58.8735, -15.975) -> (-16.1265, -15.975)
  point P0 (8.2133, 8.2133)
  dimension "d120" = 75
  dimension "d121" = 7
  dimension "d122" = 9
  dimension "d123" = 3
  measures "d120" distance between parallel lines of L5 L1
  measures "d121" distance between parallel lines of L5 L3
  measures "d122" radius of A1
  measures "d123" radius of A2
sketch "Кутник 75х8" plane through (0, 0, 0) normal (0, 0, 1) x (1, 0, 0)
  line L0 (-16.665, -16.475) -> (-16.665, 58.525)
  line L1 (-16.665, 58.525) -> (-11.665, 58.525)
  arc A0 (-8.665, 55.525) -> (-11.665, 58.525) centre (-11.665, 55.525) ccw
  line L2 (-8.665, 55.525) -> (-8.665, 0.525)
  arc A1 (-8.665, 0.525) -> (0.335, -8.475) centre (0.335, 0.525) ccw
  line L3 (0.335, -8.475) -> (55.335, -8.475)
  arc A2 (58.335, -11.475) -> (55.335, -8.475) centre (55.335, -11.475) ccw
  line L4 (58.335, -11.475) -> (58.335, -16.475)
  line L5 (58.335, -16.475) -> (-16.665, -16.475)
  point P0 (8.2133, 8.2133)
  dimension "d124" = 75
  dimension "d125" = 8
  dimension "d126" = 9
  dimension "d127" = 3
  measures "d124" distance between parallel lines of L5 L1
  measures "d125" distance between parallel lines of L5 L3
  measures "d126" radius of A1
  measures "d127" radius of A2
sketch "Кутник 75х9" plane through (0, 0, 0) normal (0, 0, 1) x (1, 0, 0)
  line L0 (-17.2035, -16.975) -> (-17.2035, 58.025)
  line L1 (-17.2035, 58.025) -> (-11.2035, 58.025)
  arc A0 (-8.2035, 55.025) -> (-11.2035, 58.025) centre (-11.2035, 55.025) ccw
  line L2 (-8.2035, 55.025) -> (-8.2035, 1.025)
  arc A1 (-8.2035, 1.025) -> (0.7965, -7.975) centre (0.7965, 1.025) ccw
  line L3 (0.7965, -7.975) -> (54.7965, -7.975)
  arc A2 (57.7965, -10.975) -> (54.7965, -7.975) centre (54.7965, -10.975) ccw
  line L4 (57.7965, -10.975) -> (57.7965, -16.975)
  line L5 (57.7965, -16.975) -> (-17.2035, -16.975)
  point P0 (8.2133, 8.2133)
  dimension "d128" = 75
  dimension "d129" = 9
  dimension "d130" = 9
  dimension "d131" = 3
  measures "d128" distance between parallel lines of L5 L1
  measures "d129" distance between parallel lines of L5 L3
  measures "d130" radius of A1
  measures "d131" radius of A2
sketch "Кутник 80х5.5" plane through (0, 0, 0) normal (0, 0, 1) x (1, 0, 0)
  line L0 (-17.2419, -17.0107) -> (-17.2419, 62.9893)
  line L1 (-17.2419, 62.9893) -> (-14.7419, 62.9893)
  arc A0 (-11.7419, 59.9893) -> (-14.7419, 62.9893) centre (-14.7419, 59.9893) ccw
  line L2 (-11.7419, 59.9893) -> (-11.7419, -2.5107)
  arc A1 (-11.7419, -2.5107) -> (-2.7419, -11.5107) centre (-2.7419, -2.5107) ccw
  line L3 (-2.7419, -11.5107) -> (59.7581, -11.5107)
  arc A2 (62.7581, -14.5107) -> (59.7581, -11.5107) centre (59.7581, -14.5107) ccw
  line L4 (62.7581, -14.5107) -> (62.7581, -17.0107)
  line L5 (62.7581, -17.0107) -> (-17.2419, -17.0107)
  point P0 (8.2133, 8.2133)
  dimension "d132" = 80
  dimension "d133" = 5.5
  dimension "d134" = 9
  dimension "d135" = 3
  measures "d132" distance between parallel lines of L5 L1
  measures "d133" distance between parallel lines of L5 L3
  measures "d134" radius of A1
  measures "d135" radius of A2
sketch "Кутник 80х6" plane through (0, 0, 0) normal (0, 0, 1) x (1, 0, 0)
  line L0 (-17.5112, -17.2607) -> (-17.5112, 62.7393)
  line L1 (-17.5112, 62.7393) -> (-14.5112, 62.7393)
  arc A0 (-11.5112, 59.7393) -> (-14.5112, 62.7393) centre (-14.5112, 59.7393) ccw
  line L2 (-11.5112, 59.7393) -> (-11.5112, -2.2607)
  arc A1 (-11.5112, -2.2607) -> (-2.5112, -11.2607) centre (-2.5112, -2.2607) ccw
  line L3 (-2.5112, -11.2607) -> (59.4888, -11.2607)
  arc A2 (62.4888, -14.2607) -> (59.4888, -11.2607) centre (59.4888, -14.2607) ccw
  line L4 (62.4888, -14.2607) -> (62.4888, -17.2607)
  line L5 (62.4888, -17.2607) -> (-17.5112, -17.2607)
  point P0 (8.2133, 8.2133)
  dimension "d136" = 80
  dimension "d137" = 6
  dimension "d138" = 9
  dimension "d139" = 3
  measures "d136" distance between parallel lines of L5 L1
  measures "d137" distance between parallel lines of L5 L3
  measures "d138" radius of A1
  measures "d139" radius of A2
sketch "Кутник 80х7" plane through (0, 0, 0) normal (0, 0, 1) x (1, 0, 0)
  line L0 (-18.0496, -17.7607) -> (-18.0496, 62.2393)
  line L1 (-18.0496, 62.2393) -> (-14.0496, 62.2393)
  arc A0 (-11.0496, 59.2393) -> (-14.0496, 62.2393) centre (-14.0496, 59.2393) ccw
  line L2 (-11.0496, 59.2393) -> (-11.0496, -1.7607)
  arc A1 (-11.0496, -1.7607) -> (-2.0496, -10.7607) centre (-2.0496, -1.7607) ccw
  line L3 (-2.0496, -10.7607) -> (58.9504, -10.7607)
  arc A2 (61.9504, -13.7607) -> (58.9504, -10.7607) centre (58.9504, -13.7607) ccw
  line L4 (61.9504, -13.7607) -> (61.9504, -17.7607)
  line L5 (61.9504, -17.7607) -> (-18.0496, -17.7607)
  point P0 (8.2133, 8.2133)
  dimension "d140" = 80
  dimension "d141" = 7
  dimension "d142" = 9
  dimension "d143" = 3
  measures "d140" distance between parallel lines of L5 L1
  measures "d141" distance between parallel lines of L5 L3
  measures "d142" radius of A1
  measures "d143" radius of A2
sketch "Кутник 80х8" plane through (0, 0, 0) normal (0, 0, 1) x (1, 0, 0)
  line L0 (-18.5881, -18.2607) -> (-18.5881, 61.7393)
  line L1 (-18.5881, 61.7393) -> (-13.5881, 61.7393)
  arc A0 (-10.5881, 58.7393) -> (-13.5881, 61.7393) centre (-13.5881, 58.7393) ccw
  line L2 (-10.5881, 58.7393) -> (-10.5881, -1.2607)
  arc A1 (-10.5881, -1.2607) -> (-1.5881, -10.2607) centre (-1.5881, -1.2607) ccw
  line L3 (-1.5881, -10.2607) -> (58.4119, -10.2607)
  arc A2 (61.4119, -13.2607) -> (58.4119, -10.2607) centre (58.4119, -13.2607) ccw
  line L4 (61.4119, -13.2607) -> (61.4119, -18.2607)
  line L5 (61.4119, -18.2607) -> (-18.5881, -18.2607)
  point P0 (8.2133, 8.2133)
  dimension "d144" = 80
  dimension "d145" = 8
  dimension "d146" = 9
  dimension "d147" = 3
  measures "d144" distance between parallel lines of L5 L1
  measures "d145" distance between parallel lines of L5 L3
  measures "d146" radius of A1
  measures "d147" radius of A2
sketch "Кутник 90х6" plane through (0, 0, 0) normal (0, 0, 1) x (1, 0, 0)
  line L0 (-21.4188, -20.8892) -> (-21.4188, 69.1108)
  line L1 (-21.4188, 69.1108) -> (-18.7188, 69.1108)
  arc A0 (-15.4188, 65.8108) -> (-18.7188, 69.1108) centre (-18.7188, 65.8108) ccw
  line L2 (-15.4188, 65.8108) -> (-15.4188, -4.8892)
  arc A1 (-15.4188, -4.8892) -> (-5.4188, -14.8892) centre (-5.4188, -4.8892) ccw
  line L3 (-5.4188, -14.8892) -> (65.2812, -14.8892)
  arc A2 (68.5812, -18.1892) -> (65.2812, -14.8892) centre (65.2812, -18.1892) ccw
  line L4 (68.5812, -18.1892) -> (68.5812, -20.8892)
  line L5 (68.5812, -20.8892) -> (-21.4188, -20.8892)
  point P0 (8.2133, 8.2133)
  dimension "d148" = 90
  dimension "d149" = 6
  dimension "d150" = 10
  dimension "d151" = 3.3
  measures "d148" distance between parallel lines of L5 L1
  measures "d149" distance between parallel lines of L5 L3
  measures "d150" radius of A1
  measures "d151" radius of A2
sketch "Кутник 90х7" plane through (0, 0, 0) normal (0, 0, 1) x (1, 0, 0)
  line L0 (-21.9573, -21.3892) -> (-21.9573, 68.6108)
  line L1 (-21.9573, 68.6108) -> (-18.2573, 68.6108)
  arc A0 (-14.9573, 65.3108) -> (-18.2573, 68.6108) centre (-18.2573, 65.3108) ccw
  line L2 (-14.9573, 65.3108) -> (-14.9573, -4.3892)
  arc A1 (-14.9573, -4.3892) -> (-4.9573, -14.3892) centre (-4.9573, -4.3892) ccw
  line L3 (-4.9573, -14.3892) -> (64.7427, -14.3892)
  arc A2 (68.0427, -17.6892) -> (64.7427, -14.3892) centre (64.7427, -17.6892) ccw
  line L4 (68.0427, -17.6892) -> (68.0427, -21.3892)
  line L5 (68.0427, -21.3892) -> (-21.9573, -21.3892)
  point P0 (8.2133, 8.2133)
  dimension "d164" = 90
  dimension "d165" = 7
  dimension "d166" = 10
  dimension "d167" = 3.3
  measures "d164" distance between parallel lines of L5 L1
  measures "d165" distance between parallel lines of L5 L3
  measures "d166" radius of A1
  measures "d167" radius of A2
sketch "Кутник 90х8" plane through (0, 0, 0) normal (0, 0, 1) x (1, 0, 0)
  line L0 (-22.4958, -21.8892) -> (-22.4958, 68.1108)
  line L1 (-22.4958, 68.1108) -> (-17.7958, 68.1108)
  arc A0 (-14.4958, 64.8108) -> (-17.7958, 68.1108) centre (-17.7958, 64.8108) ccw
  line L2 (-14.4958, 64.8108) -> (-14.4958, -3.8892)
  arc A1 (-14.4958, -3.8892) -> (-4.4958, -13.8892) centre (-4.4958, -3.8892) ccw
  line L3 (-4.4958, -13.8892) -> (64.2042, -13.8892)
  arc A2 (67.5042, -17.1892) -> (64.2042, -13.8892) centre (64.2042, -17.1892) ccw
  line L4 (67.5042, -17.1892) -> (67.5042, -21.8892)
  line L5 (67.5042, -21.8892) -> (-22.4958, -21.8892)
  point P0 (8.2133, 8.2133)
  dimension "d168" = 90
  dimension "d169" = 8
  dimension "d170" = 10
  dimension "d171" = 3.3
  measures "d168" distance between parallel lines of L5 L1
  measures "d169" distance between parallel lines of L5 L3
  measures "d170" radius of A1
  measures "d171" radius of A2
sketch "Кутник 90х9" plane through (0, 0, 0) normal (0, 0, 1) x (1, 0, 0)
  line L0 (-23.0342, -22.3892) -> (-23.0342, 67.6108)
  line L1 (-23.0342, 67.6108) -> (-17.3342, 67.6108)
  arc A0 (-14.0342, 64.3108) -> (-17.3342, 67.6108) centre (-17.3342, 64.3108) ccw
  line L2 (-14.0342, 64.3108) -> (-14.0342, -3.3892)
  arc A1 (-14.0342, -3.3892) -> (-4.0342, -13.3892) centre (-4.0342, -3.3892) ccw
  line L3 (-4.0342, -13.3892) -> (63.6658, -13.3892)
  arc A2 (66.9658, -16.6892) -> (63.6658, -13.3892) centre (63.6658, -16.6892) ccw
  line L4 (66.9658, -16.6892) -> (66.9658, -22.3892)
  line L5 (66.9658, -22.3892) -> (-23.0342, -22.3892)
  point P0 (8.2133, 8.2133)
  dimension "d172" = 90
  dimension "d173" = 9
  dimension "d174" = 10
  dimension "d175" = 3.3
  measures "d172" distance between parallel lines of L5 L1
  measures "d173" distance between parallel lines of L5 L3
  measures "d174" radius of A1
  measures "d175" radius of A2
sketch "Кутник 100х6.5" plane through (0, 0, 0) normal (0, 0, 1) x (1, 0, 0)
  line L0 (-25.6265, -24.7964) -> (-25.6265, 75.2036)
  line L1 (-25.6265, 75.2036) -> (-23.1265, 75.2036)
  arc A0 (-19.1265, 71.2036) -> (-23.1265, 75.2036) centre (-23.1265, 71.2036) ccw
  line L2 (-19.1265, 71.2036) -> (-19.1265, -6.2964)
  arc A1 (-19.1265, -6.2964) -> (-7.1265, -18.2964) centre (-7.1265, -6.2964) ccw
  line L3 (-7.1265, -18.2964) -> (70.3735, -18.2964)
  arc A2 (74.3735, -22.2964) -> (70.3735, -18.2964) centre (70.3735, -22.2964) ccw
  line L4 (74.3735, -22.2964) -> (74.3735, -24.7964)
  line L5 (74.3735, -24.7964) -> (-25.6265, -24.7964)
  point P0 (8.2133, 8.2133)
  dimension "d176" = 100
  dimension "d177" = 6.5
  dimension "d178" = 12
  dimension "d179" = 4
  measures "d176" distance between parallel lines of L5 L1
  measures "d177" distance between parallel lines of L5 L3
  measures "d178" radius of A1
  measures "d179" radius of A2
sketch "Кутник 100х7" plane through (0, 0, 0) normal (0, 0, 1) x (1, 0, 0)
  line L0 (-25.8958, -25.0464) -> (-25.8958, 74.9536)
  line L1 (-25.8958, 74.9536) -> (-22.8958, 74.9536)
  arc A0 (-18.8958, 70.9536) -> (-22.8958, 74.9536) centre (-22.8958, 70.9536) ccw
  line L2 (-18.8958, 70.9536) -> (-18.8958, -6.0464)
  arc A1 (-18.8958, -6.0464) -> (-6.8958, -18.0464) centre (-6.8958, -6.0464) ccw
  line L3 (-6.8958, -18.0464) -> (70.1042, -18.0464)
  arc A2 (74.1042, -22.0464) -> (70.1042, -18.0464) centre (70.1042, -22.0464) ccw
  line L4 (74.1042, -22.0464) -> (74.1042, -25.0464)
  line L5 (74.1042, -25.0464) -> (-25.8958, -25.0464)
  point P0 (8.2133, 8.2133)
  dimension "d180" = 100
  dimension "d181" = 7
  dimension "d182" = 12
  dimension "d183" = 4
  measures "d180" distance between parallel lines of L5 L1
  measures "d181" distance between parallel lines of L5 L3
  measures "d182" radius of A1
  measures "d183" radius of A2
sketch "Кутник 100х8" plane through (0, 0, 0) normal (0, 0, 1) x (1, 0, 0)
  line L0 (-26.4342, -25.5464) -> (-26.4342, 74.4536)
  line L1 (-26.4342, 74.4536) -> (-22.4342, 74.4536)
  arc A0 (-18.4342, 70.4536) -> (-22.4342, 74.4536) centre (-22.4342, 70.4536) ccw
  line L2 (-18.4342, 70.4536) -> (-18.4342, -5.5464)
  arc A1 (-18.4342, -5.5464) -> (-6.4342, -17.5464) centre (-6.4342, -5.5464) ccw
  line L3 (-6.4342, -17.5464) -> (69.5658, -17.5464)
  arc A2 (73.5658, -21.5464) -> (69.5658, -17.5464) centre (69.5658, -21.5464) ccw
  line L4 (73.5658, -21.5464) -> (73.5658, -25.5464)
  line L5 (73.5658, -25.5464) -> (-26.4342, -25.5464)
  point P0 (8.2133, 8.2133)
  dimension "d184" = 100
  dimension "d185" = 8
  dimension "d186" = 12
  dimension "d187" = 4
  measures "d184" distance between parallel lines of L5 L1
  measures "d185" distance between parallel lines of L5 L3
  measures "d186" radius of A1
  measures "d187" radius of A2
sketch "Кутник 100х10" plane through (0, 0, 0) normal (0, 0, 1) x (1, 0, 0)
  line L0 (-27.5112, -26.5464) -> (-27.5112, 73.4536)
  line L1 (-27.5112, 73.4536) -> (-21.5112, 73.4536)
  arc A0 (-17.5112, 69.4536) -> (-21.5112, 73.4536) centre (-21.5112, 69.4536) ccw
  line L2 (-17.5112, 69.4536) -> (-17.5112, -4.5464)
  arc A1 (-17.5112, -4.5464) -> (-5.5112, -16.5464) centre (-5.5112, -4.5464) ccw
  line L3 (-5.5112, -16.5464) -> (68.4888, -16.5464)
  arc A2 (72.4888, -20.5464) -> (68.4888, -16.5464) centre (68.4888, -20.5464) ccw
  line L4 (72.4888, -20.5464) -> (72.4888, -26.5464)
  line L5 (72.4888, -26.5464) -> (-27.5112, -26.5464)
  point P0 (8.2133, 8.2133)
  dimension "d188" = 100
  dimension "d189" = 10
  dimension "d190" = 12
  dimension "d191" = 4
  measures "d188" distance between parallel lines of L5 L1
  measures "d189" distance between parallel lines of L5 L3
  measures "d190" radius of A1
  measures "d191" radius of A2
sketch "Кутник 100х12" plane through (0, 0, 0) normal (0, 0, 1) x (1, 0, 0)
  line L0 (-28.5881, -27.5464) -> (-28.5881, 72.4536)
  line L1 (-28.5881, 72.4536) -> (-20.5881, 72.4536)
  arc A0 (-16.5881, 68.4536) -> (-20.5881, 72.4536) centre (-20.5881, 68.4536) ccw
  line L2 (-16.5881, 68.4536) -> (-16.5881, -3.5464)
  arc A1 (-16.5881, -3.5464) -> (-4.5881, -15.5464) centre (-4.5881, -3.5464) ccw
  line L3 (-4.5881, -15.5464) -> (67.4119, -15.5464)
  arc A2 (71.4119, -19.5464) -> (67.4119, -15.5464) centre (67.4119, -19.5464) ccw
  line L4 (71.4119, -19.5464) -> (71.4119, -27.5464)
  line L5 (71.4119, -27.5464) -> (-28.5881, -27.5464)
  point P0 (8.2133, 8.2133)
  dimension "d236" = 100
  dimension "d237" = 12
  dimension "d238" = 12
  dimension "d239" = 4
  measures "d236" distance between parallel lines of L5 L1
  measures "d237" distance between parallel lines of L5 L3
  measures "d238" radius of A1
  measures "d239" radius of A2
sketch "Кутник 100х14" plane through (0, 0, 0) normal (0, 0, 1) x (1, 0, 0)
  line L0 (-29.665, -28.5464) -> (-29.665, 71.4536)
  line L1 (-29.665, 71.4536) -> (-19.665, 71.4536)
  arc A0 (-15.665, 67.4536) -> (-19.665, 71.4536) centre (-19.665, 67.4536) ccw
  line L2 (-15.665, 67.4536) -> (-15.665, -2.5464)
  arc A1 (-15.665, -2.5464) -> (-3.665, -14.5464) centre (-3.665, -2.5464) ccw
  line L3 (-3.665, -14.5464) -> (66.335, -14.5464)
  arc A2 (70.335, -18.5464) -> (66.335, -14.5464) centre (66.335, -18.5464) ccw
  line L4 (70.335, -18.5464) -> (70.335, -28.5464)
  line L5 (70.335, -28.5464) -> (-29.665, -28.5464)
  point P0 (8.2133, 8.2133)
  dimension "d240" = 100
  dimension "d241" = 14
  dimension "d242" = 12
  dimension "d243" = 4
  measures "d240" distance between parallel lines of L5 L1
  measures "d241" distance between parallel lines of L5 L3
  measures "d242" radius of A1
  measures "d243" radius of A2
sketch "Кутник 100х16" plane through (0, 0, 0) normal (0, 0, 1) x (1, 0, 0)
  line L0 (-30.7419, -29.5464) -> (-30.7419, 70.4536)
  line L1 (-30.7419, 70.4536) -> (-18.7419, 70.4536)
  arc A0 (-14.7419, 66.4536) -> (-18.7419, 70.4536) centre (-18.7419, 66.4536) ccw
  line L2 (-14.7419, 66.4536) -> (-14.7419, -1.5464)
  arc A1 (-14.7419, -1.5464) -> (-2.7419, -13.5464) centre (-2.7419, -1.5464) ccw
  line L3 (-2.7419, -13.5464) -> (65.2581, -13.5464)
  arc A2 (69.2581, -17.5464) -> (65.2581, -13.5464) centre (65.2581, -17.5464) ccw
  line L4 (69.2581, -17.5464) -> (69.2581, -29.5464)
  line L5 (69.2581, -29.5464) -> (-30.7419, -29.5464)
  point P0 (8.2133, 8.2133)
  dimension "d244" = 100
  dimension "d245" = 16
  dimension "d246" = 12
  dimension "d247" = 4
  measures "d244" distance between parallel lines of L5 L1
  measures "d245" distance between parallel lines of L5 L3
  measures "d246" radius of A1
  measures "d247" radius of A2
sketch "Кутник 110х7" plane through (0, 0, 0) normal (0, 0, 1) x (1, 0, 0)
  line L0 (-29.7419, -28.6178) -> (-29.7419, 81.3822)
  line L1 (-29.7419, 81.3822) -> (-26.7419, 81.3822)
  arc A0 (-22.7419, 77.3822) -> (-26.7419, 81.3822) centre (-26.7419, 77.3822) ccw
  line L2 (-22.7419, 77.3822) -> (-22.7419, -9.6178)
  arc A1 (-22.7419, -9.6178) -> (-10.7419, -21.6178) centre (-10.7419, -9.6178) ccw
  line L3 (-10.7419, -21.6178) -> (76.2581, -21.6178)
  arc A2 (80.2581, -25.6178) -> (76.2581, -21.6178) centre (76.2581, -25.6178) ccw
  line L4 (80.2581, -25.6178) -> (80.2581, -28.6178)
  line L5 (80.2581, -28.6178) -> (-29.7419, -28.6178)
  point P0 (8.2133, 8.2133)
  dimension "d248" = 110
  dimension "d249" = 7
  dimension "d250" = 12
  dimension "d251" = 4
  measures "d248" distance between parallel lines of L5 L1
  measures "d249" distance between parallel lines of L5 L3
  measures "d250" radius of A1
  measures "d251" radius of A2
sketch "Кутник 110х8" plane through (0, 0, 0) normal (0, 0, 1) x (1, 0, 0)
  line L0 (-30.2804, -29.1178) -> (-30.2804, 80.8822)
  line L1 (-30.2804, 80.8822) -> (-26.2804, 80.8822)
  arc A0 (-22.2804, 76.8822) -> (-26.2804, 80.8822) centre (-26.2804, 76.8822) ccw
  line L2 (-22.2804, 76.8822) -> (-22.2804, -9.1178)
  arc A1 (-22.2804, -9.1178) -> (-10.2804, -21.1178) centre (-10.2804, -9.1178) ccw
  line L3 (-10.2804, -21.1178) -> (75.7196, -21.1178)
  arc A2 (79.7196, -25.1178) -> (75.7196, -21.1178) centre (75.7196, -25.1178) ccw
  line L4 (79.7196, -25.1178) -> (79.7196, -29.1178)
  line L5 (79.7196, -29.1178) -> (-30.2804, -29.1178)
  point P0 (8.2133, 8.2133)
  dimension "d256" = 110
  dimension "d257" = 8
  dimension "d258" = 12
  dimension "d259" = 4
  measures "d256" distance between parallel lines of L5 L1
  measures "d257" distance between parallel lines of L5 L3
  measures "d258" radius of A1
  measures "d259" radius of A2
sketch "Кутник 125х8" plane through (0, 0, 0) normal (0, 0, 1) x (1, 0, 0)
  line L0 (-36.1727, -34.5892) -> (-36.1727, 90.4108)
  line L1 (-36.1727, 90.4108) -> (-32.7727, 90.4108)
  arc A0 (-28.1727, 85.8108) -> (-32.7727, 90.4108) centre (-32.7727, 85.8108) ccw
  line L2 (-28.1727, 85.8108) -> (-28.1727, -12.5892)
  arc A1 (-28.1727, -12.5892) -> (-14.1727, -26.5892) centre (-14.1727, -12.5892) ccw
  line L3 (-14.1727, -26.5892) -> (84.2273, -26.5892)
  arc A2 (88.8273, -31.1892) -> (84.2273, -26.5892) centre (84.2273, -31.1892) ccw
  line L4 (88.8273, -31.1892) -> (88.8273, -34.5892)
  line L5 (88.8273, -34.5892) -> (-36.1727, -34.5892)
  point P0 (8.2133, 8.2133)
  dimension "d260" = 125
  dimension "d261" = 8
  dimension "d262" = 14
  dimension "d263" = 4.6
  measures "d260" distance between parallel lines of L5 L1
  measures "d261" distance between parallel lines of L5 L3
  measures "d262" radius of A1
  measures "d263" radius of A2
sketch "Кутник 125х9" plane through (0, 0, 0) normal (0, 0, 1) x (1, 0, 0)
  line L0 (-36.7112, -35.0892) -> (-36.7112, 89.9108)
  line L1 (-36.7112, 89.9108) -> (-32.3112, 89.9108)
  arc A0 (-27.7112, 85.3108) -> (-32.3112, 89.9108) centre (-32.3112, 85.3108) ccw
  line L2 (-27.7112, 85.3108) -> (-27.7112, -12.0892)
  arc A1 (-27.7112, -12.0892) -> (-13.7112, -26.0892) centre (-13.7112, -12.0892) ccw
  line L3 (-13.7112, -26.0892) -> (83.6888, -26.0892)
  arc A2 (88.2888, -30.6892) -> (83.6888, -26.0892) centre (83.6888, -30.6892) ccw
  line L4 (88.2888, -30.6892) -> (88.2888, -35.0892)
  line L5 (88.2888, -35.0892) -> (-36.7112, -35.0892)
  point P0 (8.2133, 8.2133)
  dimension "d264" = 125
  dimension "d265" = 9
  dimension "d266" = 14
  dimension "d267" = 4.6
  measures "d264" distance between parallel lines of L5 L1
  measures "d265" distance between parallel lines of L5 L3
  measures "d266" radius of A1
  measures "d267" radius of A2
sketch "Кутник 125х10" plane through (0, 0, 0) normal (0, 0, 1) x (1, 0, 0)
  line L0 (-37.2496, -35.5892) -> (-37.2496, 89.4108)
  line L1 (-37.2496, 89.4108) -> (-31.8496, 89.4108)
  arc A0 (-27.2496, 84.8108) -> (-31.8496, 89.4108) centre (-31.8496, 84.8108) ccw
  line L2 (-27.2496, 84.8108) -> (-27.2496, -11.5892)
  arc A1 (-27.2496, -11.5892) -> (-13.2496, -25.5892) centre (-13.2496, -11.5892) ccw
  line L3 (-13.2496, -25.5892) -> (83.1504, -25.5892)
  arc A2 (87.7504, -30.1892) -> (83.1504, -25.5892) centre (83.1504, -30.1892) ccw
  line L4 (87.7504, -30.1892) -> (87.7504, -35.5892)
  line L5 (87.7504, -35.5892) -> (-37.2496, -35.5892)
  point P0 (8.2133, 8.2133)
  dimension "d268" = 125
  dimension "d269" = 10
  dimension "d270" = 14
  dimension "d271" = 4.6
  measures "d268" distance between parallel lines of L5 L1
  measures "d269" distance between parallel lines of L5 L3
  measures "d270" radius of A1
  measures "d271" radius of A2